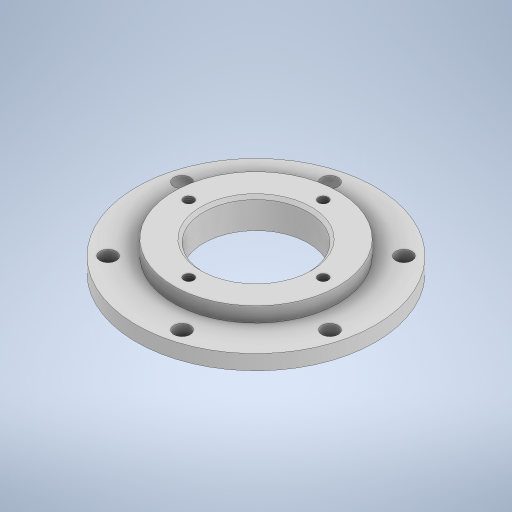
# Autodesk Inventor part: плашка
Saved by Autodesk Inventor 2023.2 (Build 272271030, 271C)
## iProperties
Created: 2024-02-27
Part Number: плашка
Material: Типовые
Document SubType Name: Modeling
Designer: user
Density: 1 g/cm^3
Appearance: По умолчанию
diam_out_plate: 160.000 mm
Author: user
Autodesk Inventor part; units mm, degrees
ref_plane "YZ Plane" through (0, 0, 0) normal (1, 0, 0) x (0, 1, 0)
ref_plane "XZ Plane" through (0, 0, 0) normal (0, 1, 0) x (-1, 0, 0)
ref_plane "XY Plane" through (0, 0, 0) normal (0, 0, 1) x (1, 0, 0)
sketch "Эскиз1" plane through (0, 0, 0) normal (0, 0, 1) x (1, 0, 0)
  line L0 (0, 0) -> (0, -30.9602)
  line L1 (35, 0) -> (35, -20)
  line L2 (35, -20) -> (80, -20)
  line L3 (80, -20) -> (80, -10)
  line L4 (80, -10) -> (55, -10)
  line L5 (55, -10) -> (55, 0)
  line L6 (55, 0) -> (35, 0)
  dimension "d0" = 70
  dimension "d1" = 110
  dimension "diam_out_plate" = 160
  dimension "d3" = 20
  dimension "d4" = 10
  constraints: 14 end point, 5 perpendicular, 2 vertical, 1 horizontal alignment
  measures "d0" diameter of L1 L0
  measures "d1" diameter of L5 L0
  measures "diam_out_plate" diameter of L3 L0
  measures "d3" distance between parallel lines of L2 L6
  measures "d4" distance between parallel lines of L2 L4
revolve "Вращение1" add sketch "Эскиз1" angle 360 about axis through (0, 0, 0) along (0, -1, 0)
sketch "Эскиз2" plane through (0, 0, 0) normal (0, 1, 0) x (1, 0, 0)
  circle A0 centre (0, 0) radius 35 projected
  circle A1 centre (0, 0) radius 55 projected
  point P0 (0, 45)
  dimension "d6" = 45
  constraints: 1 vertical alignment
  measures "d6" distance of point (0, 0) point (0, 45)
hole "Отверстие1" at (0, 0, -45) direction (0, -1, 0) diameter 6.647 depth 18 tip angle 118 thread size "M8x1.25" class "6H" standard "ISO Metric profile"
pattern_circular "Круговой массив1" count 4 over 360 about axis through (0, -10, 0) along (0, -1, 0) of "Отверстие1"
sketch "Эскиз3" plane through (0, -10, 0) normal (0, 1, 0) x (1, 0, 0)
  circle A0 centre (0, 0) radius 55 projected
  circle A1 centre (0, 0) radius 80 projected
  circle A2 centre (0, 0) radius 80 projected
  line L0 (0, 80) -> (0, 0)
  line L1 (0, 0) -> (49.4975, 49.4975) construction
  dimension "d17" = 70
  dimension "d18" = 45
  constraints: 4 end point, 1 coincident, 1 vertical, 1 vertical alignment, 1 other
  measures "d17" distance of L0.end L1.end
  measures "d18" angle of L1 L0
hole "Отверстие2" at (49.4975, -10, -49.4975) direction (0, -1, 0) diameter 11 end through all
pattern_circular "Круговой массив2" count 6 over 360 about axis through (0, -10, 0) along (0, -1, 0) of "Отверстие2"
chamfer "Фаска2" distance 2 angle 45 1 edges at (-35, 0, 0)
